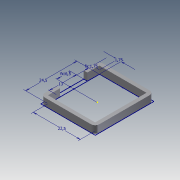
# Autodesk Inventor part: cable_tube_clip_rev1
Saved by Autodesk Inventor 2011 (Build 150239000, 239)
## iProperties
Created: 2013-02-14
Part Number: cable_tube_clip_rev1
Document SubType Name: Modeling
Designer: Administrator
Density: 1 g/cm^3
Author: Administrator
Autodesk Inventor part; units mm, degrees
ref_plane "YZ Plane" through (0, 0, 0) normal (1, 0, 0) x (0, 1, 0)
ref_plane "XZ Plane" through (0, 0, 0) normal (0, 1, 0) x (-1, 0, 0)
ref_plane "XY Plane" through (0, 0, 0) normal (0, 0, 1) x (1, 0, 0)
sketch "Sketch1" plane through (0, 0, 0) normal (0, 0, 1) x (1, 0, 0)
  line L0 (-11.25, 12.25) -> (11.25, 12.25)
  line L1 (11.25, 12.25) -> (11.25, -12.25)
  line L2 (11.25, -12.25) -> (-11.25, -12.25)
  line L3 (-11.25, -12.25) -> (-11.25, 12.25)
  line L4 (-13, 14) -> (13, 14)
  line L5 (13, 14) -> (13, -14)
  line L6 (13, -14) -> (-13, -14)
  line L7 (-13, -14) -> (-13, 14)
  line L8 (-13, 6.5) -> (-11.25, 6.5)
  line L9 (-13, -6.5) -> (-11.25, -6.5)
  point P0 (0, 0)
  point P1 (0, 12.25)
  point P2 (-11.25, 0)
  point P3 (-13, 0)
  point P4 (0, 14)
  dimension "d0" = 1.75
  dimension "d1" = 1.75
  dimension "d2" = 24.5
  dimension "d3" = 22.5
  dimension "d4" = 13
  dimension "d5" = 6.5
  constraints: 20 end point, 4 midpoint, 4 parallel, 4 perpendicular, 4 point on line, 2 horizontal, 2 horizontal alignment, 2 vertical alignment
  measures "d0" distance between parallel lines of L7 L3
  measures "d1" distance between parallel lines of L0 L4
  measures "d2" distance between parallel lines of L2 L0
  measures "d3" distance between parallel lines of L1 L3
  measures "d4" distance between parallel lines of L9 L8
  measures "d5" distance from line of point (0, 0) L8
extrude "Extrusion1" add sketch "Sketch1" along normal blind 3.5 contours L3 L8 L7 L4 L5 L6 L9 L2 L1 L0
fillet "Fillet1" radius 2 4 edges at (-13, -14, 1.75) (-13, 14, 1.75) (13, 14, 1.75) (13, -14, 1.75)
equation "\"d1\" = d0"
equation "\"d5\" = 0.5 * d4"
body "Solid1"
